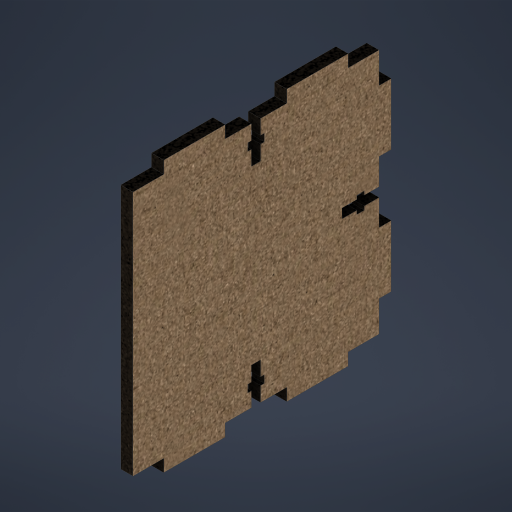
# Autodesk Inventor part: Car_Left
Saved by Autodesk Inventor 2024.1 (Build 281209000, 209)
## iProperties
Created: 2023-08-04
Part Number: Car_Left
Material: MDF Medium Density Fiberboard
Document SubType Name: Modeling
Designer: jaege
Density: 0.8 g/cm^3
Appearance: Cardboard - Corrugated
Author: jaege
Autodesk Inventor part; units mm, degrees
ref_plane "YZ Plane" through (0, 0, 0) normal (1, 0, 0) x (0, 1, 0)
ref_plane "XZ Plane" through (0, 0, 0) normal (0, 1, 0) x (-1, 0, 0)
ref_plane "XY Plane" through (0, 0, 0) normal (0, 0, 1) x (1, 0, 0)
sketch "Sketch1" plane through (0, 0, 0) normal (0, 0, 1) x (1, 0, 0)
  line L0 (0, 0) -> (0, 20) construction
  line L1 (0, 20) -> (-4, 20) projected
  line L2 (-4, 0) -> (-4, 20) projected
  line L3 (0, 0) -> (-4, 0) projected
  line L4 (0, 40) -> (0, 60) construction
  line L5 (0, 60) -> (-4, 60) projected
  line L6 (-4, 40) -> (-4, 60) projected
  line L7 (0, 40) -> (-4, 40) projected
  line L8 (0, 70) -> (-4, 70) construction
  line L9 (0, 70) -> (80, 70)
  line L10 (80, 70) -> (80, 60)
  line L11 (80, -10) -> (0, -10) construction
  line L12 (0, -10) -> (0, 0)
  line L13 (40, 70) -> (40, -10) construction
  line L14 (0, 60) -> (0, 70)
  line L15 (0, 40) -> (0, 60) construction
  line L16 (0, 20) -> (0, 40)
  line L17 (0, 0) -> (0, 20) construction
  line L18 (80, 20) -> (84, 20)
  line L19 (84, 0) -> (84, 20)
  line L20 (80, 0) -> (84, 0)
  line L21 (80, 60) -> (84, 60)
  line L22 (84, 40) -> (84, 60)
  line L23 (80, 40) -> (84, 40)
  line L24 (80, 70) -> (84, 70) construction
  line L25 (80, 60) -> (80, 40) construction
  line L26 (80, 40) -> (80, 20)
  line L27 (80, 20) -> (80, 0) construction
  line L28 (80, 0) -> (80, -10)
  line L29 (10, -10) -> (10, -14)
  line L30 (10, -14) -> (30, -14)
  line L31 (30, -10) -> (30, -14)
  line L32 (50, -10) -> (50, -14)
  line L33 (50, -14) -> (70, -14)
  line L34 (70, -10) -> (70, -14)
  line L35 (10, -10) -> (0, -10)
  line L36 (30, -10) -> (50, -10)
  line L37 (70, -10) -> (80, -10)
  point P0 (40, 30)
  dimension "d0" = 80
  dimension "d1" = 80
  dimension "d6" = 90
  constraints: 70 end point, 26 parallel, 9 symmetric about line, 5 perpendicular, 3 midpoint, 1 horizontal, 15 other
  measures "d0" distance of L11.start L11.end
  measures "d1" distance of L9.end L11.start
extrude "Extrusion1" add sketch "Sketch1" along normal blind 4
sketch "Sketch2" plane through (0, 0, 4) normal (0, 0, 1) x (1, 0, 0)
  line L0 (0, 20) -> (-4, 20) construction
  line L1 (-4, 20) -> (-4, 0) construction
  line L2 (-4, 0) -> (0, 0) construction
  line L3 (0, 0) -> (0, -10) construction
  line L4 (0, -10) -> (10, -10) construction
  line L5 (10, -10) -> (10, -14) construction
  line L6 (10, -14) -> (30, -14) construction
  line L7 (30, -14) -> (30, -10) construction
  line L8 (30, -10) -> (50, -10) construction
  line L9 (50, -10) -> (50, -14) construction
  line L10 (50, -14) -> (70, -14) construction
  line L11 (70, -14) -> (70, -10) construction
  line L12 (70, -10) -> (80, -10) construction
  line L13 (80, -10) -> (80, 0) construction
  line L14 (80, 0) -> (84, 0) construction
  line L15 (84, 0) -> (84, 20) construction
  line L16 (84, 20) -> (80, 20) construction
  line L17 (80, 20) -> (80, 40) construction
  line L18 (80, 40) -> (84, 40) construction
  line L19 (84, 40) -> (84, 60) construction
  line L20 (84, 60) -> (80, 60) construction
  line L21 (80, 60) -> (80, 70) construction
  line L22 (80, 70) -> (0, 70) construction
  line L23 (0, 70) -> (0, 60) construction
  line L24 (0, 60) -> (-4, 60) construction
  line L25 (-4, 60) -> (-4, 40) construction
  line L26 (-4, 40) -> (0, 40) construction
  line L27 (0, 40) -> (0, 20) construction
  line L28 (0, 31.5) -> (12, 31.5)
  line L29 (12, 31.5) -> (12, 28.5)
  line L30 (12, 28.5) -> (0, 28.5)
  line L31 (0, 28.5) -> (0, 31.5)
  line L32 (80, 28.5) -> (68, 28.5)
  line L33 (68, 28.5) -> (68, 31.5)
  line L34 (68, 31.5) -> (80, 31.5)
  line L35 (80, 31.5) -> (80, 28.5)
  line L36 (0, 40) -> (0, 20) projected
  line L37 (4.8, 32.7) -> (7.2, 32.7)
  line L38 (7.2, 32.7) -> (7.2, 27.3)
  line L39 (7.2, 27.3) -> (4.8, 27.3)
  line L40 (4.8, 27.3) -> (4.8, 32.7)
  line L41 (72.8, 32.7) -> (75.2, 32.7)
  line L42 (75.2, 32.7) -> (75.2, 27.3)
  line L43 (75.2, 27.3) -> (72.8, 27.3)
  line L44 (72.8, 27.3) -> (72.8, 32.7)
  line L45 (38.5, -10) -> (41.5, -10)
  line L46 (41.5, -10) -> (41.5, 2)
  line L47 (41.5, 2) -> (38.5, 2)
  line L48 (38.5, 2) -> (38.5, -10)
  line L49 (37.3, -5.2) -> (42.7, -5.2)
  line L50 (42.7, -5.2) -> (42.7, -2.8)
  line L51 (42.7, -2.8) -> (37.3, -2.8)
  line L52 (37.3, -2.8) -> (37.3, -5.2)
  line L53 (30, -10) -> (50, -10) projected
  point P0 (7.2, 30)
  point P1 (72.8, 30)
  point P2 (68, 30)
  point P3 (12, 30)
  point P4 (6, 32.7)
  point P5 (6, 31.5)
  point P6 (74, 32.7)
  point P7 (74, 31.5)
  point P8 (0, 30)
  point P9 (0, 30)
  point P10 (37.3, -4)
  point P11 (38.5, -4)
  point P12 (40, -2.8)
  point P13 (40, 2)
  point P14 (40, -10)
  point P15 (40, -10)
  point P16 (40, -10)
  point P17 (4.8, 31.5)
  point P18 (4.8, 28.5)
  point P19 (7.2, 28.5)
  point P20 (7.2, 31.5)
  point P21 (38.5, -5.2)
  point P22 (41.5, -5.2)
  point P23 (41.5, -2.8)
  point P24 (38.5, -2.8)
  point P25 (72.8, 28.5)
  point P26 (75.2, 28.5)
  point P27 (75.2, 31.5)
  point P28 (72.8, 31.5)
  dimension "d8" = 2.4
  dimension "d9" = 5.4
  dimension "d10" = 3
  dimension "d11" = 12
  constraints: 48 end point, 17 midpoint, 12 parallel, 7 equal length, 6 horizontal, 6 perpendicular, 4 horizontal alignment, 4 point on line, 3 vertical alignment, 2 coincident, 1 collinear
  measures "d8" distance of L37.start L37.end
  measures "d9" distance of L37.end L38.end
  measures "d10" distance of L28.end L29.end
  measures "d11" distance of L29.end L30.end
extrude "Extrusion2" cut sketch "Sketch2" against normal up to next
body "Solid1"
